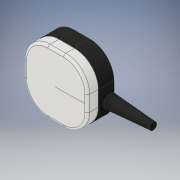
# Autodesk Inventor part: GPS_Antenna
Saved by Autodesk Inventor 2019 (Build 230136000, 136)
## iProperties
Created: 2019-04-19
Part Number: GPS_Antenna
Material: Generic
Document SubType Name: Modeling
Designer: CASE-SMALL2
Density: 1 g/cm^3
Appearance: Default
Author: CASE-SMALL2
Autodesk Inventor part; units mm, degrees
ref_plane "YZ Plane" through (0, 0, 0) normal (1, 0, 0) x (0, 1, 0)
ref_plane "XZ Plane" through (0, 0, 0) normal (0, 1, 0) x (-1, 0, 0)
ref_plane "XY Plane" through (0, 0, 0) normal (0, 0, 1) x (1, 0, 0)
sketch "Sketch1" plane through (0, 0, 0) normal (0, 0, 1) x (1, 0, 0)
  line L0 (-26.5, -26.5) -> (26.5, -26.5)
  line L1 (26.5, -26.5) -> (26.5, 26.5)
  line L2 (26.5, 26.5) -> (-26.5, 26.5)
  line L3 (-26.5, 26.5) -> (-26.5, -26.5)
  line L4 (-26.5, -26.5) -> (26.5, 26.5) construction
  line L5 (26.5, -26.5) -> (-26.5, 26.5) construction
  point P0 (0, 0)
  dimension "d0" = 53
  dimension "d1" = 53
  constraints: 12 end point, 2 midpoint, 2 parallel, 1 horizontal, 1 perpendicular
  measures "d0" distance of L1.end L2.end
  measures "d1" distance of L0.end L1.end
extrude "Extrusion1" add sketch "Sketch1" along normal blind 12.8
fillet "Fillet1" radius 20 4 edges at (-26.5, -26.5, 6.4) (26.5, -26.5, 6.4) (26.5, 26.5, 6.4) (-26.5, 26.5, 6.4)
sketch "Sketch3" plane through (0, 0, 12.8) normal (0, 0, 1) x (1, 0, 0)
  arc A0 (-6.5, 26.5) -> (-26.5, 6.5) centre (-6.5, 6.5) ccw projected
  line L0 (-26.5, 6.5) -> (-26.5, -6.5) projected
  arc A1 (-26.5, -6.5) -> (-6.5, -26.5) centre (-6.5, -6.5) ccw projected
  line L1 (-6.5, -26.5) -> (6.5, -26.5) projected
  arc A2 (6.5, -26.5) -> (26.5, -6.5) centre (6.5, -6.5) ccw projected
  line L2 (26.5, -6.5) -> (26.5, 6.5) projected
  arc A3 (26.5, 6.5) -> (6.5, 26.5) centre (6.5, 6.5) ccw projected
  line L3 (6.5, 26.5) -> (-6.5, 26.5) projected
  arc A4 (6.5, -26.2) -> (26.2, -6.5) centre (6.5, -6.5) ccw
  line L4 (6.5, -26.2) -> (-6.5, -26.2)
  arc A5 (-26.2, -6.5) -> (-6.5, -26.2) centre (-6.5, -6.5) ccw
  line L5 (-26.2, -6.5) -> (-26.2, 6.5)
  arc A6 (-6.5, 26.2) -> (-26.2, 6.5) centre (-6.5, 6.5) ccw
  line L6 (-6.5, 26.2) -> (6.5, 26.2)
  arc A7 (26.2, 6.5) -> (6.5, 26.2) centre (6.5, 6.5) ccw
  line L7 (26.2, 6.5) -> (26.2, -6.5)
  point P0 (0, 0)
  dimension "d5" = 0.3
  constraints: 8 end point, 8 point on circle, 4 centre point, 7 other
  measures "d5" distance between parallel lines of L1 L4
extrude "Extrusion2" add sketch "Sketch3" along normal blind 9.8 separate body contours L4 A5 L5 A6 L6 A7 L7 A4
sketch "Sketch4" plane through (0, 0, 0) normal (0, 1, 0) x (-1, 0, 0)
  line L0 (-6.5, 22.6) -> (6.5, 22.6) construction
  line L1 (0, 22.4946) -> (-8.086, 22.4517) construction
  line L2 (-8.086, 22.4517) -> (-14.4882, 22.4967) construction
  line L3 (-14.4882, 22.4967) -> (-34.2, 21.6) construction
  spline S0 degree 3 poles (0, 22.4946) (-8.086, 22.4517) (-14.4882, 22.4967) (-34.2, 21.6) knots 1 1 1 1 2 2 2 2
  line L4 (-26.2, 12.8) -> (-26.2, 22.6) construction
  line L5 (0, -4.5801) -> (0, 27.4806) projected
  line L6 (0, 22.4946) -> (0, 22.6)
  line L7 (0, 22.6) -> (-34.2, 22.6)
  line L8 (-34.2, 22.6) -> (-34.2, 21.6)
  point P0 (0, 0)
  point P1 (-26.5, 0)
  dimension "d8" = 21.6
  dimension "d10" = 8
  constraints: 6 end point, 2 point on line, 1 midpoint, 1 perpendicular, 3 other
  measures "d8" vertical distance of point (-26.5, 0) L3.end
  measures "d10" distance from line of L4 L3.end
revolve "Revolution1" cut sketch "Sketch4" angle 360 about axis through (0, 0, -10) along (0, 0, 1) bodies 2
fillet "Fillet2" radius 2 9 edges at (26.2, -3.2272, 21.9347) (20.4267, -20.4333, 21.8325) (0.0314, -26.2, 21.9425) (-20.4387, -20.4213, 21.8325) (-26.2, -0.0314, 21.9425) (-20.4265, 20.4335, 21.8325) (-0.0314, 26.2, 21.9425) (20.4335, 20.4265, 21.8325) (26.2, 3.293, 21.9343)
sketch "Sketch5" plane through (26.5, -6.5, 0) normal (1, 0, 0) x (0, 0, -1)
  circle A0 centre (-3.5, 0) radius 5.5
  line L0 (0, 0) -> (0, 13) projected
  line L1 (4.96, 6.5) -> (-15.76, 6.5) projected
  point P0 (0, 6.5)
  dimension "d12" = 11
  dimension "d13" = 3.5
  dimension "d14" = 6.5
  constraints: 1 centre point
  measures "d12" diameter of A0
  measures "d13" distance from line of L0 A0.centre
  measures "d14" distance from line of L1 A0.centre
extrude "Extrusion3" add sketch "Sketch5" along normal blind 36 bodies 1
chamfer "Chamfer1" distance 35.25 angle 4 1 edges at (62.5, -6.5, 9) measured on face at (50.5, -1.1581, 2.1909)
sketch "Sketch6" plane through (0, 0, 0) normal (0, 0, -1) x (-1, 0, 0)
  circle A0 centre (0, 0) radius 2
  circle A1 centre (19.25, 19.25) radius 1.15
  line L0 (0, -42.7993) -> (0, 42.7993) projected
  line L1 (49.1851, 0) -> (-81.1142, 0) projected
  circle A2 centre (19.25, -19.25) radius 1.15
  circle A3 centre (-19.25, 19.25) radius 1.15
  circle A4 centre (-19.25, -19.25) radius 1.15
  dimension "d20" = 4
  dimension "d21" = 2.3
  dimension "d23" = 18.1
  dimension "d25" = 18.1
  constraints: 5 centre point, 3 symmetric about line, 1 coincident, 3 other
  measures "d20" diameter of A0
  measures "d21" diameter of A1
  measures "d23" distance edge to line of A1 L1
  measures "d25" distance edge to line of A1 L0
extrude "Extrusion4" cut sketch "Sketch6" against normal blind 6 bodies 1
sketch "Sketch7" plane through (0, 0, 0) normal (0, 0, -1) x (-1, 0, 0)
  line L0 (47.219, 0) -> (-80.7865, 0) construction
  line L1 (0, -40.5055) -> (0, 40.5055) construction
  circle A0 centre (22.5, 0) radius 3.25
  circle A1 centre (0, 22.5) radius 3.25
  line L2 (26.5, 6.5) -> (26.5, -6.5) projected
  line L3 (-6.5, 26.5) -> (6.5, 26.5) projected
  line L4 (-47.219, 0) -> (80.7865, 0) construction
  circle A2 centre (-22.5, 0) radius 3.25
  line L5 (0, 40.5055) -> (0, -40.5055) construction
  circle A3 centre (0, -22.5) radius 3.25
  point P0 (0, 0)
  dimension "d28" = 6.5
  dimension "d29" = 4
  dimension "d30" = 4
  dimension "d31" = 6.5
  constraints: 6 symmetric about line, 4 centre point, 4 end point, 4 point on line, 2 other
  measures "d28" diameter of A0
  measures "d29" distance from line of L2 A0.centre
  measures "d30" distance from line of L3 A1.centre
  measures "d31" diameter of A1
extrude "Extrusion5" cut sketch "Sketch7" against normal blind 6 bodies 1
sketch "Sketch8" plane through (-22.5, 0, 6) normal (0, 0, -1) x (-1, 0, 0)
  circle A0 centre (0, 0) radius 3.25 projected
  circle A1 centre (-22.5, 22.5) radius 3.25 projected
  circle A2 centre (-45, 0) radius 3.25 projected
  circle A3 centre (-22.5, -22.5) radius 3.25 projected
  point P0 (-22.5, 0)
extrude "Extrusion6" add sketch "Sketch8" along normal blind 6 separate body
equation "\"d1\" = d0"
equation "\"d25\" = d23"
equation "\"d30\" = d29"
equation "\"d31\" = d28"
body "Solid1"
body "Solid2"
body "Solid3"
